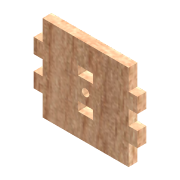
# Autodesk Inventor part: joystick binnenkant
Saved by Autodesk Inventor 2020.3 (Build 243373000, 373)
## iProperties
Created: 2020-12-09
Part Number: joystick binnenkant
Material: Wood (Birch)
Document SubType Name: Sheet Metal
Designer: Svend
Density: 0.55 g/cm^3
Sheet Metal Rule: Default_mm
Appearance: Birch - Natural Polished
Author: Svend
Autodesk Inventor part; units mm, degrees
ref_plane "YZ Plane" through (0, 0, 0) normal (1, 0, 0) x (0, 1, 0)
ref_plane "XZ Plane" through (0, 0, 0) normal (0, 1, 0) x (-1, 0, 0)
ref_plane "XY Plane" through (0, 0, 0) normal (0, 0, 1) x (1, 0, 0)
ref_plane "Work Plane1" through (0, 0, 0) normal (0, 0, 1) x (1, 0, 0)
sketch "Sketch1" plane through (0, 0, 0) normal (0, 0, 1) x (1, 0, 0)
  line L0 (-10, 0) -> (-10, 6)
  line L1 (-10, 6) -> (-34, 6)
  line L2 (-34, 0) -> (-34, 6)
  line L3 (-34, 0) -> (-10, 0)
  line L4 (-10, 21) -> (-10, 27)
  line L5 (-10, 27) -> (-34, 27)
  line L6 (-34, 21) -> (-34, 27)
  line L7 (-34, 21) -> (-10, 21)
  line L8 (0, 21) -> (0, 27)
  line L9 (0, 21) -> (24, 21)
  line L10 (24, 21) -> (24, 27)
  line L11 (24, 27) -> (0, 27)
  line L12 (0, 0) -> (0, 6)
  line L13 (0, 0) -> (24, 0)
  line L14 (24, 0) -> (24, 6)
  line L15 (24, 6) -> (0, 6)
  line L16 (24, 8.5) -> (30, 8.5)
  line L17 (30, 8.5) -> (30, -1.5)
  line L18 (24, -1.5) -> (30, -1.5)
  line L19 (24, -1.5) -> (24, 8.5)
  line L20 (24, 18.5) -> (30, 18.5)
  line L21 (24, 18.5) -> (24, 28.5)
  line L22 (24, 28.5) -> (30, 28.5)
  line L23 (30, 28.5) -> (30, 18.5)
  line L24 (10, -15.5) -> (20, -15.5)
  line L25 (24, -11.5) -> (24, -1.5)
  line L26 (24, 28.5) -> (24, 38.5)
  line L27 (20, 42.5) -> (10, 42.5)
  line L28 (-20, 42.5) -> (-30, 42.5)
  line L29 (-34, 38.5) -> (-34, 28.5)
  line L30 (-34, 8.5) -> (-34, 18.5)
  line L31 (-34, -11.5) -> (-34, -1.5)
  line L32 (-30, -15.5) -> (-20, -15.5)
  line L33 (-10, -15.5) -> (0, -15.5)
  line L34 (10, -15.5) -> (20, -15.5)
  line L35 (-34, -15.5) -> (24, -15.5)
  line L36 (24, -15.5) -> (24, 42.5)
  line L37 (24, 42.5) -> (-34, 42.5)
  line L38 (-34, 42.5) -> (-34, -15.5)
  line L39 (-34, 8.5) -> (-40, 8.5)
  line L40 (-34, 8.5) -> (-34, -1.5)
  line L41 (-34, -1.5) -> (-40, -1.5)
  line L42 (-40, -1.5) -> (-40, 8.5)
  line L43 (-34, 18.5) -> (-40, 18.5)
  line L44 (-40, 18.5) -> (-40, 28.5)
  line L45 (-34, 28.5) -> (-40, 28.5)
  line L46 (-34, 28.5) -> (-34, 18.5)
  line L47 (0, 27) -> (-10, 27)
  line L48 (-10, 21) -> (-10, 27)
  line L49 (-10, 21) -> (0, 21)
  line L50 (0, 21) -> (0, 27)
  line L51 (0, 6) -> (-10, 6)
  line L52 (-10, 0) -> (-10, 6)
  line L53 (-10, 0) -> (0, 0)
  line L54 (0, 0) -> (0, 6)
extrude "Plate1" add sketch "Sketch1" along normal blind 6 contours L3 L2 L1 L0 | L53 L13 L19 L25 L36 L35 L24 L33 L32 L38 L31 L3 | L1 L38 L30 L7 L49 L9 L21 L36 L19 L15 L51 | L38 L41 L42 L39 L2 | L12 L15 L14 L13 | L14 L19 L16 L17 L18 | L43 L44 L45 L38 L6 | L6 L5 L4 L7 | L21 L10 L22 L23 L20 | L38 L29 L37 L28 L27 L36 L26 L21 L11 L47 L5 | L9 L8 L11 L10
sketch "Sketch2" plane through (0, 0, 6) normal (0, 0, 1) x (1, 0, 0)
  line L0 (-10, 27) -> (0, 27) projected
  line L1 (0, 27) -> (0, 21) projected
  line L2 (0, 21) -> (-10, 21) projected
  line L3 (-10, 21) -> (-10, 27) projected
  line L4 (0, 0) -> (-10, 0) projected
  line L5 (-10, 0) -> (-10, 6) projected
  line L6 (-10, 6) -> (0, 6) projected
  line L7 (0, 6) -> (0, 0) projected
  line L8 (30, -1.5) -> (24, -1.5) projected
  line L9 (30, 8.5) -> (30, -1.5) projected
  line L10 (24, 8.5) -> (30, 8.5) projected
  line L11 (24, 18.5) -> (24, 8.5) projected
  line L12 (30, 18.5) -> (24, 18.5) projected
  line L13 (30, 28.5) -> (30, 18.5) projected
  line L14 (24, 28.5) -> (30, 28.5) projected
  line L15 (24, 42.5) -> (24, 28.5) projected
  line L16 (-34, 42.5) -> (24, 42.5) projected
  line L17 (-34, 28.5) -> (-34, 42.5) projected
  line L18 (-40, 28.5) -> (-34, 28.5) projected
  line L19 (-40, 18.5) -> (-40, 28.5) projected
  line L20 (-34, 18.5) -> (-40, 18.5) projected
  line L21 (-34, 8.5) -> (-34, 18.5) projected
  line L22 (-40, 8.5) -> (-34, 8.5) projected
  line L23 (-40, -1.5) -> (-40, 8.5) projected
  line L24 (-34, -1.5) -> (-40, -1.5) projected
  line L25 (-34, -15.5) -> (-34, -1.5) projected
  line L26 (24, -15.5) -> (-34, -15.5) projected
  line L27 (24, -1.5) -> (24, -15.5) projected
  circle A0 centre (-5, 13.5) radius 2.5
  point P0 (0, 0)
  point P1 (-5, 6)
  point P2 (-34, 13.5)
  dimension "d1" = 5
  constraints: 2 midpoint, 1 centre point, 1 horizontal alignment, 1 vertical alignment
  measures "d1" diameter of A0
extrude "Cut1" cut sketch "Sketch2" against normal blind 6 contours A0
equation "\"d2\" = Thickness"
equation "\"d0\" = Thickness"
equation "\"BendRadius\" = Thickness"
equation "\"BendReliefWidth\" = Thickness"
equation "\"BendReliefDepth\" = 0.5 * Thickness"
equation "\"CornerReliefSize\" = 4 * Thickness"
equation "\"MinimumRemnant\" = 2 * Thickness"
equation "\"TransitionRadius\" = BendRadius"
equation "\"JacobiRadiusSize\" = BendRadius"
equation "\"GapSize\" = Thickness"
equation "\"Thickness\" = 6"
body "Solid1"
